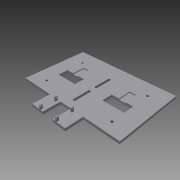
# Autodesk Inventor part: Top
Saved by Autodesk Inventor 2015 (Build 190159000, 159)
## iProperties
Created: 2018-12-21
Part Number: Top
Material: Типовые
Document SubType Name: Modeling
Designer: kostya
Density: 1 g/cm^3
Appearance: По умолчанию
Author: kostya
Autodesk Inventor part; units mm, degrees
ref_plane "YZ Plane" through (0, 0, 0) normal (1, 0, 0) x (0, 1, 0)
ref_plane "XZ Plane" through (0, 0, 0) normal (0, 1, 0) x (-1, 0, 0)
ref_plane "XY Plane" through (0, 0, 0) normal (0, 0, 1) x (1, 0, 0)
sketch "Эскиз1" plane through (0, 0, 0) normal (0, 0, 1) x (1, 0, 0)
  line L0 (-100, -75) -> (100, -75)
  line L1 (100, -75) -> (100, 75)
  line L2 (100, 75) -> (-100, 75)
  line L3 (-100, 75) -> (-100, -75)
  line L4 (-100, -75) -> (100, 75) construction
  line L5 (100, -75) -> (-100, 75) construction
  point P0 (0, 0)
  dimension "d0" = 200
  dimension "d1" = 150
  constraints: 12 end point, 2 midpoint, 2 parallel, 1 horizontal, 1 perpendicular
  measures "d0" distance of L2.end L1.end
  measures "d1" distance of L1.end L0.end
extrude "Выдавливание1" add sketch "Эскиз1" along normal blind 5
sketch "Эскиз2" plane through (0, 0, 5) normal (0, 0, 1) x (1, 0, 0)
  line L0 (100, -75) -> (100, 75) construction
  line L1 (100, 0) -> (-100, 0) construction
  line L2 (-100, 75) -> (-100, -75) construction
  line L3 (100, 75) -> (-100, 75) construction
  line L4 (0, 75) -> (0, -75) construction
  line L5 (-100, -75) -> (100, -75) construction
  line L6 (-100, -10) -> (100, -10) construction
  line L7 (100, -10) -> (100, 10) construction
  line L8 (100, 10) -> (-100, 10) construction
  line L9 (-100, 10) -> (-100, -10) construction
  line L10 (-100, -10) -> (100, 10) construction
  line L11 (100, -10) -> (-100, 10) construction
  line L12 (0, 0) -> (-100, 0) construction
  line L13 (-50, 0) -> (-50, 75) construction
  line L14 (0, 0) -> (100, 0) construction
  line L15 (50, 0) -> (50, 75) construction
  line L16 (-56, 10) -> (-56, 35)
  line L17 (-56, 35) -> (-44, 35)
  line L18 (-44, 35) -> (-44, 10)
  line L19 (-56, 10) -> (-44, 10)
  line L20 (56, 10) -> (56, 35)
  line L21 (56, 35) -> (44, 35)
  line L22 (44, 35) -> (44, 10)
  line L23 (56, 10) -> (44, 10)
  line L24 (-70, -10) -> (-30, -10)
  line L25 (-30, -10) -> (-30, 10)
  line L26 (-30, 10) -> (-70, 10)
  line L27 (-70, 10) -> (-70, -10)
  line L28 (-70, -10) -> (-30, 10) construction
  line L29 (-30, -10) -> (-70, 10) construction
  line L30 (70, -10) -> (30, -10)
  line L31 (30, -10) -> (30, 10)
  line L32 (30, 10) -> (70, 10)
  line L33 (70, 10) -> (70, -10)
  dimension "d4" = 20
  dimension "d7" = 25
  dimension "d8" = 40
  constraints: 60 end point, 10 midpoint, 8 symmetric about line, 7 perpendicular, 6 point on line, 4 parallel, 2 collinear, 2 horizontal, 1 vertical
  measures "d4" distance of L7.end L6.end
  measures "d7" distance of L16.start L16.end
  measures "d8" distance of L26.end L25.end
extrude "Выдавливание2" cut sketch "Эскиз2" against normal blind 2 contours L16 L17 L18 L19 | L23 L22 L21 L20
extrude "Выдавливание3" cut sketch "Эскиз2" against normal blind 5 contours L19 L26 L25 L24 L27 | L32 L33 L30 L31 L23
sketch "Эскиз3" plane through (0, 0, 3) normal (0, 0, 1) x (1, 0, 0)
  line L0 (-56, 10) -> (-56, 35) projected
  line L1 (-44, 10) -> (-56, 10) projected
  line L2 (-44, 35) -> (-44, 10) projected
  line L3 (-56, 35) -> (-44, 35) projected
  line L4 (-44, 35) -> (-44, 10) projected
  point P0 (0, 0)
surface extrude "ВыдавПврх1" sketch "Эскиз3" along normal blind 10 shown no curves L4 L1 L0 L3
boundary_patch "Участок поверхности1"
sketch "Эскиз4" plane through (-56, 10, 3) normal (0, -1, 0) x (1, 0, 0)
  line L0 (0, 10) -> (12, 10) construction
  line L1 (6, 10) -> (6, 0) construction
  line L2 (12, 0) -> (0, 0) construction
  line L3 (0, 0) -> (0, 10) construction
  line L4 (0, 5) -> (12, 5) construction
  line L5 (12, 0) -> (12, 10) construction
  arc A0 (7.118, 4) -> (4.882, 4) centre (6, 5) ccw
  line L6 (6, 3.5) -> (6, 4) construction
  line L7 (6, 4) -> (7.118, 4)
  line L8 (6, 4) -> (4.882, 4)
  point P0 (56, -3)
  dimension "d17" = 3
  dimension "d18" = 0.5
  constraints: 10 end point, 5 midpoint, 2 point on circle, 2 point on line, 1 centre point, 1 horizontal, 1 perpendicular
  measures "d17" diameter of A0
  measures "d18" distance of L6.start L6.end
surface extrude "ВыдавПврх2" sketch "Эскиз4" along normal blind 10 shown no curves L7 A0 L8
boundary_patch "Участок поверхности2"
mirror "Зеркальное отражение1" [suppressed]
ref_plane "РабПлоскость1" through (-70, 0, 5) normal (0, -1, 0) x (1, 0, 0)
sketch "Эскиз6" plane through (0, 0, 5) normal (0, 0, 1) x (1, 0, 0)
  line L0 (-100, -75) -> (100, -75) projected
  line L1 (100, -75) -> (100, 75) projected
  line L2 (100, 75) -> (-100, 75) projected
  line L3 (-100, 75) -> (-100, -75) projected
  line L4 (-44, 10) -> (-30, 10) projected
  line L5 (-30, 10) -> (-30, -10) projected
  line L6 (-30, -10) -> (-70, -10) projected
  line L7 (-70, -10) -> (-70, 10) projected
  line L8 (-70, 10) -> (-56, 10) projected
  line L9 (-56, 10) -> (-56, 35) projected
  line L10 (-56, 35) -> (-44, 35) projected
  line L11 (-44, 35) -> (-44, 10) projected
  line L12 (30, 10) -> (44, 10) projected
  line L13 (44, 10) -> (44, 35) projected
  line L14 (44, 35) -> (56, 35) projected
  line L15 (56, 35) -> (56, 10) projected
  line L16 (56, 10) -> (70, 10) projected
  line L17 (70, 10) -> (70, -10) projected
  line L18 (70, -10) -> (30, -10) projected
  line L19 (30, -10) -> (30, 10) projected
  line L20 (100, -75) -> (70, -75)
  line L21 (100, -45) -> (100, -75)
  line L22 (-100, 0) -> (100, 0) construction
  line L23 (100, 75) -> (-100, 75) construction
  line L24 (0, 75) -> (0, -75) construction
  circle A0 centre (70, 45) radius 2.5
  line L25 (70, 45) -> (70, 75) construction
  line L26 (70, 45) -> (100, 45) construction
  line L27 (100, -75) -> (100, 75) projected
  line L28 (100, 10) -> (70, 10) construction
  line L29 (70, 10) -> (70, -10) construction
  line L30 (70, -10) -> (100, -10) construction
  line L31 (100, -10) -> (100, 10) construction
  line L32 (70, -75) -> (70, -35) construction
  line L33 (70, -75) -> (110, -75) construction
  line L34 (70, -35) -> (100, -35) construction
  circle A1 centre (70, -35) radius 2.5
  circle A2 centre (-70, 45) radius 2.5
  line L35 (-70, 45) -> (-70, 75) construction
  line L36 (-70, 45) -> (-100, 45) construction
  line L37 (-70, -75) -> (-70, -35) construction
  line L38 (-70, -35) -> (-100, -35) construction
  circle A3 centre (-70, -35) radius 2.5
  line L39 (100, -75) -> (100, -55)
  line L40 (100, -55) -> (-100, -55)
  point P0 (0, 0)
  dimension "d39" = 30
  dimension "d40" = 30
  dimension "d41" = 40
  dimension "d42" = 90
  dimension "d43" = 5
  dimension "d44" = 20
  constraints: 38 end point, 8 symmetric about line, 6 point on line, 4 centre point, 4 coincident, 4 midpoint, 4 perpendicular, 3 horizontal, 2 parallel, 1 vertical, 2 other
  measures "d39" distance of L25.start L25.end
  measures "d40" distance of L25.start L26.end
  measures "d41" distance of L20.end L32.end
  measures "d42" angle of L33 L32
  measures "d43" diameter of A1
  measures "d44" distance of L0.end L39.end
extrude "Выдавливание5" cut sketch "Эскиз6" against normal blind 10 contours A0 | A1 | A2 | A3
sketch "Эскиз7" plane through (0, 0, 5) normal (0, 0, 1) x (1, 0, 0)
  line L0 (-100, -75) -> (100, -75) projected
  line L1 (100, -75) -> (100, 75) projected
  line L2 (100, 75) -> (-100, 75) projected
  line L3 (-100, 75) -> (-100, -75) projected
  line L4 (-44, 10) -> (-30, 10) projected
  line L5 (-30, 10) -> (-30, -10) projected
  line L6 (-30, -10) -> (-70, -10) projected
  line L7 (-70, -10) -> (-70, 10) projected
  line L8 (-70, 10) -> (-56, 10) projected
  line L9 (-56, 10) -> (-56, 35) projected
  line L10 (-56, 35) -> (-44, 35) projected
  line L11 (-44, 35) -> (-44, 10) projected
  line L12 (30, 10) -> (44, 10) projected
  line L13 (44, 10) -> (44, 35) projected
  line L14 (44, 35) -> (56, 35) projected
  line L15 (56, 35) -> (56, 10) projected
  line L16 (56, 10) -> (70, 10) projected
  line L17 (70, 10) -> (70, -10) projected
  line L18 (70, -10) -> (30, -10) projected
  line L19 (30, -10) -> (30, 10) projected
  line L20 (100, 75) -> (-100, 75) construction
  line L21 (-30, 10) -> (30, 10) construction
  line L22 (30, 10) -> (30, 75) construction
  line L23 (30, 75) -> (-30, 75) construction
  line L24 (-30, 75) -> (-30, 10) construction
  line L25 (-100, -75) -> (100, -75) construction
  line L26 (-30, -10) -> (30, -10) construction
  line L27 (30, -10) -> (30, -75) construction
  line L28 (30, -75) -> (-30, -75) construction
  line L29 (-30, -75) -> (-30, -10) construction
  line L30 (100, -75) -> (100, 75) construction
  line L31 (100, -7.5) -> (100, 7.5) construction
  line L32 (100, 7.5) -> (-100, 7.5) construction
  line L33 (-100, 7.5) -> (-100, -7.5) construction
  line L34 (-100, -7.5) -> (100, 7.5) construction
  line L35 (100, -7.5) -> (-100, 7.5) construction
  line L36 (-100, -7.5) -> (-2.5, -7.5) construction
  line L37 (2.5, -7.5) -> (100, -7.5) construction
  line L38 (-100, 75) -> (-100, -75) construction
  line L39 (-100, 0) -> (100, 0) construction
  arc A0 (-2.5, 7.5) -> (2.5, 7.5) centre (0, 7.5) ccw
  line L40 (2.5, 7.5) -> (2.5, 38.1)
  line L41 (-2.5, 38.1) -> (-2.5, 7.5)
  arc A1 (2.5, 38.1) -> (-2.5, 38.1) centre (0, 38.1) ccw
  line L42 (-2.5, 38.1) -> (-2.5, 7.5)
  line L43 (2.5, 7.5) -> (2.5, 38.1)
  line L44 (-2.5, -38.1) -> (-2.5, -7.5)
  line L45 (2.5, -7.5) -> (2.5, -38.1)
  arc A2 (-2.5, -38.1) -> (2.5, -38.1) centre (0, -38.1) ccw
  arc A3 (2.5, -7.5) -> (-2.5, -7.5) centre (0, -7.5) ccw
  point P0 (0, 0)
  dimension "d31" = 15
  constraints: 44 end point, 8 parallel, 8 point on circle, 6 symmetric about line, 4 centre point, 4 horizontal, 4 midpoint, 4 perpendicular, 4 point on line, 1 collinear, 1 other
  measures "d31" distance of L31.end L31.start
extrude "Выдавливание7" cut sketch "Эскиз7" against normal blind 10 contours L41 A1 L40 A0 | L44 A3 L45 A2
extrude "Выдавливание8" cut sketch "Эскиз6" against normal blind 10 contours L3 L40 L1 L0
sketch "Эскиз13" plane through (0, 0, 5) normal (0, 0, 1) x (1, 0, 0)
  line L0 (-100, -55) -> (100, -55) projected
  line L1 (100, -55) -> (100, 75) projected
  line L2 (100, 75) -> (-100, 75) projected
  line L3 (-100, 75) -> (-100, -55) projected
  line L4 (30, 10) -> (44, 10) projected
  line L5 (44, 10) -> (44, 35) projected
  line L6 (44, 35) -> (56, 35) projected
  line L7 (56, 35) -> (56, 10) projected
  line L8 (56, 10) -> (70, 10) projected
  line L9 (70, 10) -> (70, -10) projected
  line L10 (70, -10) -> (30, -10) projected
  line L11 (30, -10) -> (30, 10) projected
  line L12 (-44, 10) -> (-30, 10) projected
  line L13 (-30, 10) -> (-30, -10) projected
  line L14 (-30, -10) -> (-70, -10) projected
  line L15 (-70, -10) -> (-70, 10) projected
  line L16 (-70, 10) -> (-56, 10) projected
  line L17 (-56, 10) -> (-56, 35) projected
  line L18 (-56, 35) -> (-44, 35) projected
  line L19 (-44, 35) -> (-44, 10) projected
  circle A0 centre (-70, -35) radius 2.5 projected
  circle A1 centre (70, -35) radius 2.5 projected
  circle A2 centre (70, 45) radius 2.5 projected
  circle A3 centre (-70, 45) radius 2.5 projected
  arc A4 (2.5, -7.5) -> (-2.5, -7.5) centre (0, -7.5) ccw projected
  line L20 (2.5, -7.5) -> (2.5, -38.1) projected
  arc A5 (-2.5, -38.1) -> (2.5, -38.1) centre (0, -38.1) ccw projected
  line L21 (-2.5, -38.1) -> (-2.5, -7.5) projected
  arc A6 (-2.5, 7.5) -> (2.5, 7.5) centre (0, 7.5) ccw projected
  line L22 (-2.5, 7.5) -> (-2.5, 38.1) projected
  arc A7 (2.5, 38.1) -> (-2.5, 38.1) centre (0, 38.1) ccw projected
  line L23 (2.5, 38.1) -> (2.5, 7.5) projected
  line L24 (0, 75) -> (0, -55) construction
  point P0 (0, 0)
  constraints: 2 end point, 1 midpoint, 1 vertical
sketch "Эскиз14" plane through (0, 0, 5) normal (0, 0, 1) x (1, 0, 0)
  line L0 (-100, -55) -> (100, -55) projected
  line L1 (5, -55) -> (35, -55)
  line L2 (5, -55) -> (12, -55)
  line L3 (12, -55) -> (35, -55)
  line L4 (35, -55) -> (35, -87) construction
  line L5 (35, -87) -> (12, -87) construction
  line L6 (12, -87) -> (12, -55) construction
  line L7 (12, -71) -> (35, -71) construction
  line L8 (23.5, -55) -> (23.5, -87) construction
  line L9 (12, -55) -> (11, -55) construction
  line L10 (36, -87) -> (11, -87)
  line L11 (11, -87) -> (11, -55)
  line L12 (11, -55) -> (36, -55)
  line L13 (36, -55) -> (36, -87)
  line L14 (36, -87) -> (11, -55) construction
  line L15 (11, -87) -> (36, -55) construction
  arc A0 (-2.5, -38.1) -> (2.5, -38.1) centre (0, -38.1) ccw projected
  line L16 (0, -40.6) -> (5, -40.6) construction
  line L17 (0, -40.6) -> (-5, -40.6) construction
  line L18 (0, -40.6) -> (0, -67.546) construction
  line L19 (100, -55) -> (-100, -55)
  line L20 (-5, -55) -> (-35, -55)
  line L21 (-5, -55) -> (-12, -55)
  line L22 (-12, -55) -> (-35, -55)
  line L23 (-35, -55) -> (-35, -87) construction
  line L24 (-35, -87) -> (-12, -87) construction
  line L25 (-12, -87) -> (-12, -55) construction
  line L26 (-12, -71) -> (-35, -71) construction
  line L27 (-23.5, -55) -> (-23.5, -87) construction
  line L28 (-12, -55) -> (-11, -55) construction
  line L29 (-36, -87) -> (-11, -87)
  line L30 (-11, -87) -> (-11, -55)
  line L31 (-11, -55) -> (-36, -55)
  line L32 (-36, -55) -> (-36, -87)
  line L33 (-36, -87) -> (-11, -55) construction
  line L34 (-11, -87) -> (-36, -55) construction
  point P0 (0, 0)
  dimension "d70" = 30
  dimension "d71" = 7
  dimension "d72" = 32
  dimension "d73" = 1
  dimension "d103" = 5
  dimension "d104" = 5
  constraints: 68 end point, 16 symmetric about line, 4 horizontal, 4 midpoint, 4 parallel, 4 point on line, 2 perpendicular, 2 tangent, 1 point on circle, 1 vertical
  measures "d70" distance of L1.start L1.end
  measures "d71" distance of L1.start L2.end
  measures "d72" distance of L3.end L4.end
  measures "d73" distance of L2.end L9.end
  measures "d103" distance of L16.start L16.end
  measures "d104" distance of L16.start L17.end
extrude "Выдавливание12" add sketch "Эскиз14" against normal up to surface (5 mm away)
sketch "Эскиз15" plane through (0, 0, 5) normal (0, 0, 1) x (1, 0, 0)
  line L0 (30, 10) -> (44, 10) projected
  line L1 (44, 10) -> (44, 35) projected
  line L2 (44, 35) -> (56, 35) projected
  line L3 (56, 35) -> (56, 10) projected
  line L4 (56, 10) -> (70, 10) projected
  line L5 (70, 10) -> (70, -10) projected
  line L6 (70, -10) -> (30, -10) projected
  line L7 (30, -10) -> (30, 10) projected
  line L8 (-44, 10) -> (-30, 10) projected
  line L9 (-30, 10) -> (-30, -10) projected
  line L10 (-30, -10) -> (-70, -10) projected
  line L11 (-70, -10) -> (-70, 10) projected
  line L12 (-70, 10) -> (-56, 10) projected
  line L13 (-56, 10) -> (-56, 35) projected
  line L14 (-56, 35) -> (-44, 35) projected
  line L15 (-44, 35) -> (-44, 10) projected
  line L16 (-100, -55) -> (-36, -55) projected
  line L17 (11, -55) -> (11, -87) projected
  line L18 (11, -87) -> (36, -87) projected
  line L19 (36, -87) -> (36, -55) projected
  line L20 (36, -55) -> (100, -55) projected
  line L21 (100, -55) -> (100, 75) projected
  line L22 (100, 75) -> (-100, 75) projected
  line L23 (-100, 75) -> (-100, -55) projected
  circle A0 centre (-70, -35) radius 2.5 projected
  circle A1 centre (70, -35) radius 2.5 projected
  circle A2 centre (70, 45) radius 2.5 projected
  circle A3 centre (-70, 45) radius 2.5 projected
  arc A4 (2.5, -7.5) -> (-2.5, -7.5) centre (0, -7.5) ccw projected
  line L24 (2.5, -7.5) -> (2.5, -38.1) projected
  arc A5 (-2.5, -38.1) -> (2.5, -38.1) centre (0, -38.1) ccw projected
  line L25 (-2.5, -38.1) -> (-2.5, -7.5) projected
  arc A6 (-2.5, 7.5) -> (2.5, 7.5) centre (0, 7.5) ccw projected
  line L26 (-2.5, 7.5) -> (-2.5, 38.1) projected
  arc A7 (2.5, 38.1) -> (-2.5, 38.1) centre (0, 38.1) ccw projected
  line L27 (2.5, 38.1) -> (2.5, 7.5) projected
  line L28 (11, -87) -> (16.3, -87)
  line L29 (16.3, -87) -> (16.3, -82.6)
  line L30 (16.3, -87) -> (18.7, -87)
  line L31 (18.7, -87) -> (18.7, -82.6)
  line L32 (18.7, -82.6) -> (16.3, -82.6)
  line L33 (11, -55) -> (11, -55.8)
  line L34 (11, -55.8) -> (36, -55.8) construction
  line L35 (11, -55.8) -> (16.3, -55.8) construction
  line L36 (16.3, -55.8) -> (16.3, -60.2)
  line L37 (16.3, -60.2) -> (18.7, -60.2)
  line L38 (18.7, -60.2) -> (18.7, -55.8)
  line L39 (16.3, -55.8) -> (18.7, -55.8)
  line L40 (-36, -55) -> (-36, -87) projected
  line L41 (-36, -87) -> (-11, -87) projected
  line L42 (-11, -87) -> (-11, -55) projected
  line L43 (-11, -55) -> (11, -55) projected
  arc A8 (-2.5, -38.1) -> (2.5, -38.1) centre (0, -38.1) ccw construction
  line L44 (0, -40.6) -> (0, -65.8945) construction
  line L45 (-11, -87) -> (-36, -87)
  line L46 (-11, -87) -> (-16.3, -87)
  line L47 (-16.3, -87) -> (-16.3, -82.6)
  line L48 (-16.3, -87) -> (-18.7, -87)
  line L49 (-18.7, -87) -> (-18.7, -82.6)
  line L50 (-18.7, -82.6) -> (-16.3, -82.6)
  line L51 (-11, -55.8) -> (-36, -55.8) construction
  line L52 (-11, -55.8) -> (-16.3, -55.8) construction
  line L53 (-16.3, -55.8) -> (-16.3, -60.2)
  line L54 (-16.3, -60.2) -> (-18.7, -60.2)
  line L55 (-18.7, -60.2) -> (-18.7, -55.8)
  line L56 (-16.3, -55.8) -> (-18.7, -55.8)
  point P0 (0, 0)
  dimension "d77" = 5.3
  dimension "d78" = 4.4
  dimension "d79" = 2.4
  dimension "d80" = 0.8
  dimension "d81" = 5.3
  dimension "d82" = 4.4
  constraints: 50 end point, 10 point on line, 10 symmetric about line, 3 perpendicular, 3 vertical, 2 horizontal, 2 point on circle, 1 collinear
  measures "d77" distance of L17.end L28.end
  measures "d78" distance of L28.end L29.end
  measures "d79" distance of L28.end L30.end
  measures "d80" distance of L17.start L33.end
  measures "d81" distance of L33.end L35.end
  measures "d82" distance of L35.end L36.end
extrude "Выдавливание13" add sketch "Эскиз15" along normal blind 8 contours L49 L50 L47 L41 | L18 L29 L32 L31 | L39 L38 L37 L36 | L53 L54 L55 L56
sketch "Эскиз16" plane through (16.3, -87, 5) normal (-1, 0, 0) x (0, 0, 1)
  line L0 (0, 0) -> (0, 4.4) projected
  line L1 (0, 0) -> (8, 0) projected
  line L2 (8, 4.4) -> (8, 0) projected
  line L3 (0, 4.4) -> (8, 4.4) projected
  line L4 (0, 0) -> (5.5, 0)
  line L5 (5.5, 0) -> (5.5, 1.81)
  line L6 (0, 0) -> (8, 0) projected
  line L7 (5.4488, 0) -> (5.5, 0)
  line L8 (6.4488, 0) -> (6.4488, 1.81)
  line L9 (6.4488, 1.81) -> (5.9488, 2.2999) construction
  arc A0 (6.4488, 1.81) -> (5.5, 1.7627) centre (5.9488, 2.2999) ccw
  point P0 (-5, 87)
  dimension "d85" = 5.5
  dimension "d86" = 1.81
  dimension "d87" = 1
  dimension "d88" = 0.7
  constraints: 10 end point, 4 point on line, 2 point on circle, 1 centre point, 1 coincident, 1 perpendicular, 1 vertical
  measures "d85" distance of L4.end L0.start
  measures "d86" distance of L4.end L5.end
  measures "d87" distance of L7.start L8.start
  measures "d88" distance of L8.end L9.end
extrude "Выдавливание14" cut sketch "Эскиз16" against normal blind 8 contours L5 A0 L8 L1
ref_plane "РабПлоскость5" through (16.3, -71.4, 5) normal (0, -1, 0) x (1, 0, 0)
mirror "Зеркальное отражение4" about plane through (16.3, -71.4, 5) normal (0, -1, 0) of "Выдавливание14"
ref_plane "РабПлоскость6" through (23.5, -87, 5) normal (1, 0, 0) x (0, 0, -1)
sketch "Эскиз19" plane through (0, 0, 5) normal (0, 0, 1) x (1, 0, 0)
  circle A0 centre (70, 45) radius 2.5 projected
  circle A1 centre (70, -35) radius 2.5 projected
  line L0 (30, 10) -> (44, 10) projected
  line L1 (44, 10) -> (44, 35) projected
  line L2 (44, 35) -> (56, 35) projected
  line L3 (56, 35) -> (56, 10) projected
  line L4 (56, 10) -> (70, 10) projected
  line L5 (70, 10) -> (70, -10) projected
  line L6 (70, -10) -> (30, -10) projected
  line L7 (30, -10) -> (30, 10) projected
  arc A2 (-2.5, 7.5) -> (2.5, 7.5) centre (0, 7.5) ccw projected
  line L8 (-2.5, 7.5) -> (-2.5, 38.1) projected
  arc A3 (2.5, 38.1) -> (-2.5, 38.1) centre (0, 38.1) ccw projected
  line L9 (2.5, 38.1) -> (2.5, 7.5) projected
  arc A4 (2.5, -7.5) -> (-2.5, -7.5) centre (0, -7.5) ccw projected
  line L10 (2.5, -7.5) -> (2.5, -38.1) projected
  arc A5 (-2.5, -38.1) -> (2.5, -38.1) centre (0, -38.1) ccw projected
  line L11 (-2.5, -38.1) -> (-2.5, -7.5) projected
  circle A6 centre (-70, 45) radius 2.5 projected
  circle A7 centre (-70, -35) radius 2.5 projected
  line L12 (-44, 10) -> (-30, 10) projected
  line L13 (-30, 10) -> (-30, -10) projected
  line L14 (-30, -10) -> (-70, -10) projected
  line L15 (-70, -10) -> (-70, 10) projected
  line L16 (-70, 10) -> (-56, 10) projected
  line L17 (-56, 10) -> (-56, 35) projected
  line L18 (-56, 35) -> (-44, 35) projected
  line L19 (-44, 35) -> (-44, 10) projected
  line L20 (16.3, -55.8) -> (18.7, -55.8) projected
  line L21 (18.7, -55.8) -> (18.7, -60.2) projected
  line L22 (18.7, -60.2) -> (16.3, -60.2) projected
  line L23 (16.3, -60.2) -> (16.3, -55.8) projected
  line L24 (18.7, -87) -> (36, -87) projected
  line L25 (36, -87) -> (36, -55) projected
  line L26 (36, -55) -> (100, -55) projected
  line L27 (100, -55) -> (100, 75) projected
  line L28 (100, 75) -> (-100, 75) projected
  line L29 (-100, 75) -> (-100, -55) projected
  line L30 (11, -55) -> (11, -87) projected
  line L31 (11, -87) -> (16.3, -87) projected
  line L32 (16.3, -87) -> (16.3, -82.6) projected
  line L33 (16.3, -82.6) -> (18.7, -82.6) projected
  line L34 (18.7, -82.6) -> (18.7, -87) projected
  line L35 (-70, -35) -> (-70, -55) construction
  line L36 (70, -35) -> (70, -55) construction
  line L37 (36, -55) -> (100, -55) construction
  line L38 (-70, -55) -> (-60, -55) construction
  line L39 (-60, -55) -> (-55, -55)
  line L40 (-55, -55) -> (-55, -50)
  line L41 (-55, -50) -> (-60, -50)
  line L42 (-60, -50) -> (-60, -55)
  line L43 (-36, -55) -> (-36, -87) projected
  line L44 (-16.3, -87) -> (-11, -87) projected
  line L45 (-11, -87) -> (-11, -55) projected
  line L46 (-11, -55) -> (11, -55) projected
  line L47 (-18.7, -87) -> (-18.7, -82.6) projected
  line L48 (-18.7, -82.6) -> (-16.3, -82.6) projected
  line L49 (-16.3, -82.6) -> (-16.3, -87) projected
  line L50 (-100, -55) -> (-36, -55) projected
  line L51 (-36, -87) -> (-18.7, -87) projected
  point P0 (0, 0)
  dimension "d100" = 10
  dimension "d101" = 5
  dimension "d102" = 5
  constraints: 14 end point, 2 parallel, 2 perpendicular, 1 horizontal, 1 point on line, 1 vertical
  measures "d100" distance of L35.end L38.end
  measures "d101" distance of L41.end L40.end
  measures "d102" distance of L40.end L39.end
ref_plane "РабПлоскость7" through (0, -87, 5) normal (1, 0, 0) x (0, 0, -1)
mirror "Зеркальное отражение5" about plane through (0, -87, 5) normal (1, 0, 0) of "Выдавливание14", "Зеркальное отражение4"
body "SRF1"
body "SRF2"
body "SRF3"
body "SRF4"
body "SRF5"
body "SRF6"
body "SRF7"
